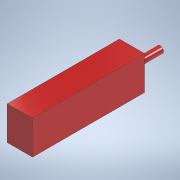
# Autodesk Inventor part: czesc3
Saved by Autodesk Inventor 2022 (Build 260153000, 153)
## iProperties
Created: 2022-06-07
Part Number: czesc3
Material: Ogólny
Document SubType Name: Sheet Metal
Designer: admin
Density: 1 g/cm^3
Sheet Metal Rule: Domyślny_mm
Appearance: Domyślna
Author: admin
Autodesk Inventor part; units mm, degrees
ref_plane "YZ Plane" through (0, 0, 0) normal (1, 0, 0) x (0, 1, 0)
ref_plane "XZ Plane" through (0, 0, 0) normal (0, 1, 0) x (-1, 0, 0)
ref_plane "XY Plane" through (0, 0, 0) normal (0, 0, 1) x (1, 0, 0)
sketch "Szkic1" plane through (0, 0, 0) normal (0, 1, 0) x (-1, 0, 0)
  line L0 (45, 200) -> (-45, 200)
  line L1 (-45, 200) -> (-45, -200)
  line L2 (-45, -200) -> (45, -200)
  line L3 (45, -200) -> (45, 200)
  line L4 (45, 200) -> (-45, -200) construction
  line L5 (-45, 200) -> (45, -200) construction
  point P0 (0, 0)
  dimension "d0" = 90
  dimension "d1" = 400
  constraints: 12 end point, 2 midpoint, 2 parallel, 1 horizontal, 1 perpendicular
  measures "d0" distance of L2.end L1.end
  measures "d1" distance of L1.end L0.end
extrude "Wyciągnięcie proste1" add sketch "Szkic1" along normal blind 120
sketch "Szkic2" plane through (45, 0, -200) normal (0, 0, -1) x (-1, 0, 0)
  line L0 (90, 0) -> (90, 120) projected
  line L1 (0, 0) -> (90, 0) projected
  line L2 (0, 0) -> (0, 120) projected
  line L3 (0, 120) -> (90, 120) projected
  circle A0 centre (45, 60) radius 12.5
  point P0 (45, 0)
  dimension "d4" = 25
  dimension "d5" = 60
  dimension "d6" = 45
  constraints: 1 centre point
  measures "d4" diameter of A0
  measures "d5" distance from line of L1 A0.centre
  measures "d6" distance from line of L2 A0.centre
extrude "Wyciągnięcie proste2" add sketch "Szkic2" along normal blind 100 contours A0
equation "\"PromieńGięcia\" = Grubość"
equation "\"SzerokośćGięciaPodcięcia\" = Grubość"
equation "\"GłębokośćGięciaPodcięcia\" = 0.5 * Grubość"
equation "\"RozmiarPodcięciaNarożnika\" = 4 * Grubość"
equation "\"MinimalnaPozostałość\" = 2 * Grubość"
equation "\"PromieńPrzejścia\" = PromieńGięcia"
equation "\"Rozmiar_promienia_Jacobiego\" = PromieńGięcia"
equation "\"Wielk_odstępu\" = Grubość"
equation "\"Grubość\" = 0.5"
